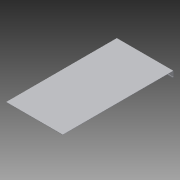
# Autodesk Inventor part: workTable
Saved by Autodesk Inventor 2013 (Build 170138000, 138)
## iProperties
Created: 2012-10-22
Part Number: workTable
Material: Aluminum 6061
Document SubType Name: Sheet Metal
Designer: Istvan
Density: 2.71 g/cm^3
Sheet Metal Rule: Default
Author: Istvan
Autodesk Inventor part; units mm, degrees
ref_plane "YZ Plane" through (0, 0, 0) normal (1, 0, 0) x (0, 1, 0)
ref_plane "XZ Plane" through (0, 0, 0) normal (0, 1, 0) x (-1, 0, 0)
ref_plane "XY Plane" through (0, 0, 0) normal (0, 0, 1) x (1, 0, 0)
sketch "Sketch1" plane through (0, 0, 0) normal (0, 1, 0) x (-1, 0, 0)
  line L0 (0, 0) -> (546.1, 0)
  line L1 (546.1, 0) -> (546.1, 1066.8)
  line L2 (546.1, 1066.8) -> (0, 1066.8)
  line L3 (0, 1066.8) -> (0, 0)
  dimension "d0" = 546.1
  dimension "d1" = 1066.8
  measures "d0" distance of L2.end L1.end
  measures "d1" distance of L1.end L0.end
extrude "Plate1" add sketch "Sketch1" along normal blind 3.048
sketch "Sketch2" plane through (0, -3.048, -3.048) normal (0, 0, -1) x (-1, 0, 0)
  line L0 (546.1, 0) -> (0, 0)
  line L1 (0, 0) -> (0, -57.404)
  line L2 (0, -57.404) -> (546.1, -57.404)
  line L3 (546.1, -57.404) -> (546.1, 0)
  constraints: 6 end point, 1 horizontal, 1 perpendicular, 1 vertical
edge flange "Flange1" height 63.5 angle 90 thickness 3.048 bend radius 3.048 thickness toward (0, 0, -1) relief straight relief width 3.048 relief depth 1.524 edges at (-273.05, 0, 0) wall of the first edge with corners at (-546.1, -3.048, -3.048) (0, -3.048, -3.048) (0, -60.452, -3.048) (-546.1, -60.452, -3.048)
bend "Bend1"
corner "Corner1"
sketch "Sketch3" plane through (-546.1, -56.642, -3.048) normal (-1, 0, 0) x (0, -1, 0)
  line L0 (0, -3.048) -> (0, 0)
  arc A0 (0, 0) -> (0, 1.524) centre (0, 0.762) ccw
  line L1 (0, 1.524) -> (-8.382, 1.524)
  line L2 (-8.382, 1.524) -> (-8.382, 4.572)
  line L3 (-8.382, 4.572) -> (0, 4.572)
  arc A1 (0, -3.048) -> (0, 4.572) centre (0, 0.762) ccw
  constraints: 8 end point, 4 point on circle
hem "Hem1" sketch "Sketch3" thickness 3.048 along (1, 0, 0) edges at (-273.05, -60.452, -3.048)
equation "\"d13\" = BendReliefWidth"
equation "\"d14\" = BendReliefDepth"
equation "\"d15\" = MinimumRemnant"
equation "\"d16\" = BendRadius"
equation "\"d17\" = 4 * Thickness"
equation "\"d18\" = 0.5 * Thickness"
equation "\"d19\" = 0.5 * d18"
equation "\"d3\" = BendReliefWidth"
equation "\"d4\" = BendReliefDepth"
equation "\"d5\" = MinimumRemnant"
equation "\"d6\" = BendRadius"
equation "\"d9\" = BendRadius"
equation "\"d10\" = CornerReliefSize"
equation "\"d11\" = GapSize"
equation "\"d12\" = JacobiRadiusSize"
equation "\"BendRadius\" = Thickness"
equation "\"BendReliefWidth\" = Thickness"
equation "\"BendReliefDepth\" = 0.5 * Thickness"
equation "\"CornerReliefSize\" = 4 * Thickness"
equation "\"MinimumRemnant\" = 2 * Thickness"
equation "\"TransitionRadius\" = BendRadius"
equation "\"JacobiRadiusSize\" = BendRadius"
equation "\"GapSize\" = Thickness"
equation "\"d2\" = BendRadius"
equation "\"Thickness\" = 3.048"
body "Solid1"
